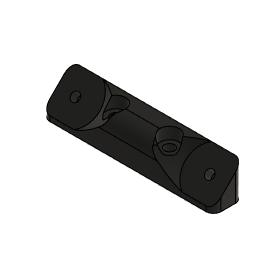
PredatorCarriageAdapterForHaydnMagball (Autodesk Fusion 360 design; units mm, degrees)
Autodesk Fusion 360 part; units mm, degrees
sketch "Sketch1" plane through (0, 0, 0) normal (0, 0, 1) x (1, 0, 0)
  line L0 (0, 0) -> (11, 0) construction
  circle A0 centre (11, 0) radius 2.1
  line L1 (0, 0) -> (0, -6) construction
  line L2 (0, -6) -> (35, -6)
  line L3 (35, -6) -> (35, 6)
  line L4 (35, 6) -> (0, 6)
  line L5 (0, 6) -> (0, -6)
  circle A1 centre (11, 0) radius 4
  dimension "d1" = 11
  dimension "d2" = 4.2
  dimension "d3" = 6
  dimension "d4" = 35
  dimension "d5" = 12
  dimension "d6" = 8
  constraint coincident L0.start L1.start
  constraint horizontal L0
  constraint coincident L0.end A0.centre
  constraint perpendicular L0 L1
  constraint horizontal L2
  constraint vertical L3
  constraint horizontal L4
  constraint vertical L5
  constraint concentric A0 A1
  measures "d1" distance of L0.start L0.end
  measures "d2" diameter of A0
  measures "d3" distance of L0.start L1.end
  measures "d4" distance of L1.end L2.end
  measures "d5" distance of L1.end L4.end
  measures "d6" diameter of A1
extrude "Extrude1" add sketch "Sketch1" along normal blind 14 contours L2 L3 L4 L5 makes body 1
extrude "Extrude2" add sketch "Sketch1" along normal blind 9.2 contours A1 bodies 1
ref_plane "WorkPlane1" through (17.5, 6, 14) normal (0, -0.707107, 0.707107) x (-1, 0, 0)
sketch "Sketch2" plane through (17.5, 6, 14) normal (0, -0.707107, 0.707107) x (-1, 0, 0)
  line L0 (17.5, 0) -> (-10, 0) construction
  line L1 (-10, 0) -> (-10, 8.5) construction
  line L2 (-4.7322, 0) -> (-17.5, 0)
  line L3 (-17.5, 0) -> (-17.5, 17)
  line L4 (-17.5, 17) -> (-4.7322, 17)
  arc A0 (-4.7322, 0) -> (-4.7322, 17) centre (-10, 8.5) ccw
  circle A1 centre (-10, 8.5) radius 1.8
  line L5 (-12.75, 6.9123) -> (-10, 5.3246)
  line L6 (-10, 5.3246) -> (-7.25, 6.9123)
  line L7 (-7.25, 6.9123) -> (-7.25, 10.0877)
  line L8 (-7.25, 10.0877) -> (-10, 11.6754)
  line L9 (-10, 11.6754) -> (-12.75, 10.0877)
  line L10 (-12.75, 10.0877) -> (-12.75, 6.9123)
  point P0 (-10, 8.5)
  dimension "d12" = 27.5
  dimension "d13" = 8.5
  dimension "d17" = 3.6
  dimension "d20" = 2.75
  constraint horizontal L0
  constraint perpendicular L0 L1
  constraint coincident P0 L1.end
  constraint coincident L0 L2.start
  constraint perpendicular L1 L2
  constraint perpendicular L0 L3
  constraint perpendicular L3 L4
  constraint concentric A0 A1
  measures "d12" distance of L0.start L0.end
  measures "d13" distance of L0.end P0
  measures "d17" diameter of A1
  measures "d20" distance of P0 L10
extrude "Extrude3" cut sketch "Sketch2" along normal blind 8.5 contours L2 L3 L4 A0 | A1 | L5 L6 L7 L8 L9 L10 bodies 1
extrude "Extrude4" cut sketch "Sketch2" against normal blind 10 contours A1 bodies 1
extrude "Extrude5" cut sketch "Sketch2" against normal blind 6 from surface at -4 contours L5 L6 L7 L8 L9 L10 bodies 1
ref_plane "WorkPlane3" through (26.2423, -9.8995, 17.8995) normal (0, -0.707107, 0.707107) x (-1, 0, 0)
sketch "Sketch3" plane through (26.2423, -9.8995, 17.8995) normal (0, -0.707107, 0.707107) x (-1, 0, 0)
  line L0 (26.2425, 0) -> (-1.2575, 0) construction
  circle A0 centre (-1.2575, 0) radius 30
  dimension "d30" = 27.5
  dimension "d31" = 60
  constraint horizontal L0
  constraint coincident L0.end A0.centre
  measures "d30" distance of L0.start L0.end
  measures "d31" diameter of A0
loft "Loft2" cut profiles "Sketch2", "Sketch3" section 1 contours L2 L3 L4 A0 section 2 bodies 1
fillet "Fillet2" radius 3 2 edges at (35, -6, 1) (35, 6, 7) on bodies 1
mirror "Mirror2" about plane through (0, 0, 0) normal (1, 0, 0) of bodies 1 makes body 2
combine "Combine2" operation add target body 1 tool bodies 2
sketch "Sketch4" plane through (0, 6, 0) normal (0, 1, 0) x (-1, 0, 0)
  line L0 (-32, 14) -> (-32, 0)
  line L1 (-32, 0) -> (-30.25, 0)
  line L2 (-30.25, 0) -> (-30.25, 4.2246)
  line L3 (-30.25, 4.2246) -> (-27.5, 6.4699)
  line L4 (-27.5, 6.4699) -> (-24.75, 4.2246)
  line L5 (-24.75, 4.2246) -> (-24.75, 0)
  line L6 (-24.75, 0) -> (24.75, 0)
  line L7 (24.75, 0) -> (24.75, 4.2246)
  line L8 (24.75, 4.2246) -> (27.5, 6.4699)
  line L9 (27.5, 6.4699) -> (30.25, 4.2246)
  line L10 (30.25, 4.2246) -> (30.25, 0)
  line L11 (30.25, 0) -> (32, 0)
  line L12 (32, 0) -> (32, 14)
  line L13 (32, 14) -> (22.2322, 14)
  line L14 (22.2322, 14) -> (-22.2322, 14)
  line L15 (-22.2322, 14) -> (-32, 14)
  line L16 (0, 0) -> (0, 10) construction
  line L17 (0, 0) -> (0, 2.5) construction
  line L18 (0, 2.5) -> (-4, 2.5) construction
  line L19 (-4, 2.5) -> (-9, 2.5) construction
  point P0 (-4, 2.5)
  dimension "d35" = 2.5
  dimension "d36" = 4
  dimension "d37" = 5
  constraint coincident L16.start L17.start
  constraint perpendicular L6 L16
  constraint perpendicular L6 L17
  constraint perpendicular L16 L18
  constraint parallel L18 L19
  constraint coincident P0 L18.end
  measures "d35" distance of L16.start L17.end
  measures "d36" distance of L17.end P0
  measures "d37" distance of P0 L19.end
hole "Hole1" at (0, 6, 10) direction (0, -1, 0) diameter 3.332 depth 8 tip angle 118 bodies 1
thread "Thread1" "ISO Metric profile 4.0 M4x0.7 6H"
hole "Hole2" at (9, 6, 2.5) at (4, 6, 2.5) direction (0, -1, 0) diameter 1.623 depth 6 tip angle 118 bodies 1
thread "Thread2" "ISO Metric profile 2.0 M2x0.4 6H"
fillet "Fillet3" radius 6 3 edges at (0, -6, 14) (-6.9201, -4.5008, 14) (6.9201, -4.5008, 14) on bodies 1
equation "d9 = 14 mm - 4.8 mm"
equation "d12 = ( 55 / 2 ) * 1 mm"
equation "d13 = ( 17 / 2 ) * 1 mm"
equation "d20 = ( 5.5 / 2 ) * 1 mm"
named bodies: "Body2"
